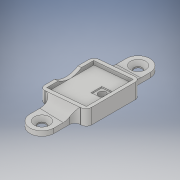
# Autodesk Inventor part: Kamerahalterung_Winkel_variabel
Saved by Autodesk Inventor 2019 (Build 230136000, 136)
## iProperties
Created: 2020-05-14
Part Number: Kamerahalterung_Winkel_variabel
Material: Generisch
Document SubType Name: Modeling
Designer: 111162002
Density: 1 g/cm^3
Appearance: Vorgabe
Author: 111162002
Autodesk Inventor part; units mm, degrees
ref_plane "YZ Plane" through (0, 0, 0) normal (1, 0, 0) x (0, 1, 0)
ref_plane "XZ Plane" through (0, 0, 0) normal (0, 1, 0) x (-1, 0, 0)
ref_plane "XY Plane" through (0, 0, 0) normal (0, 0, 1) x (1, 0, 0)
sketch "Skizze2" plane through (0, 0, 0) normal (0, 0, 1) x (1, 0, 0)
  line L0 (0, 0) -> (0, 9.3)
  line L1 (0, 9.3) -> (39, 12.7121)
  line L2 (39, 12.7121) -> (39, 0)
  line L3 (39, 0) -> (0, 0)
  dimension "d0" = 95
  dimension "d1" = 9.3
  dimension "d5" = 39
  constraints: 8 end point, 1 parallel, 1 perpendicular, 1 vertical
  measures "d0" angle of L1 L0
  measures "d1" distance of L0.start L0.end
  measures "d5" horizontal distance of L1.end L0.end
extrude "Extrusion1" add sketch "Skizze2" along normal blind 45
sketch "Skizze3" plane through (0, 9.3, 45) normal (-0.0871557, 0.9961947, 0) x (0.9961947, 0.0871557, 0)
  line L0 (3.0245, 42) -> (36.1245, 42)
  line L1 (36.1245, 42) -> (36.1245, 3)
  line L2 (36.1245, 3) -> (3.0245, 3)
  line L3 (3.0245, 3) -> (3.0245, 42)
  line L4 (39.149, 0) -> (0, 0) projected
  line L5 (39.149, 45) -> (39.149, 0) projected
  line L6 (33.249, 27.8623) -> (23.749, 27.8623)
  line L7 (23.749, 27.8623) -> (23.749, 18.8623)
  line L8 (23.749, 18.8623) -> (33.249, 18.8623)
  line L9 (33.249, 18.8623) -> (33.249, 27.8623)
  circle A0 centre (28.499, 23.3623) radius 3
  point P0 (-0.8105, 45)
  dimension "d6" = 39
  dimension "d7" = 33.1
  dimension "d8" = 3
  dimension "d9" = 3.0245
  dimension "d10" = 9
  dimension "d11" = 9.5
  dimension "d12" = 5.9
  dimension "d13" = 6
  dimension "d14" = 4.75
  constraints: 16 end point, 4 parallel, 2 horizontal, 2 perpendicular, 1 centre point
  measures "d6" distance of L0.end L1.end
  measures "d7" distance of L0.start L0.end
  measures "d8" distance between parallel lines of L4 L2
  measures "d9" distance between parallel lines of L5 L1
  measures "d10" distance of L6.end L7.end
  measures "d11" distance of L7.end L8.end
  measures "d12" distance between parallel lines of L5 L9
  measures "d13" diameter of A0
  measures "d14" distance from line of A0.centre L9
extrude "Extrusion2" cut sketch "Skizze3" against normal blind 3 contours L0 L1 L2 L3
extrude "Extrusion3" cut sketch "Skizze3" against normal up to surface contours A0 surface through (0, 0, 0) normal (0, -1, 0)
extrude "Extrusion4" cut sketch "Skizze3" against normal blind 4 contours L9 L8 L7 L6
sketch "Skizze5" plane through (0, 0, 0) normal (0, -1, 0) x (1, 0, 0)
  line L0 (39, 0) -> (0, 0) projected
  line L1 (9.5, 0) -> (29.5, 0)
  line L2 (29.5, 0) -> (29.5, -27.5)
  line L3 (29.5, -27.5) -> (9.5, -27.5)
  line L4 (9.5, -27.5) -> (9.5, 0)
  line L5 (0, 0) -> (0, 45) projected
  line L6 (0, 45) -> (39, 45) projected
  line L7 (9.5, 45) -> (29.5, 45)
  line L8 (29.5, 45) -> (29.5, 72.5)
  line L9 (29.5, 72.5) -> (9.5, 72.5)
  line L10 (9.5, 72.5) -> (9.5, 45)
  circle A0 centre (19.5, -17.5) radius 3.25
  circle A1 centre (19.5, 62.5) radius 3.25
  dimension "d26" = 20
  dimension "d27" = 9.5
  dimension "d28" = 27.5
  dimension "d29" = 27.5
  dimension "d30" = 20
  dimension "d32" = 9.5
  dimension "d35" = 6.5
  dimension "d36" = 6.5
  dimension "d37" = 10
  dimension "d38" = 10
  dimension "d39" = 10
  dimension "d40" = 10
  constraints: 16 end point, 4 parallel, 2 centre point, 2 horizontal, 2 perpendicular, 2 point on line
  measures "d26" distance of L2.end L3.end
  measures "d27" distance between parallel lines of L5 L4
  measures "d28" distance of L3.end L1.start
  measures "d29" distance of L9.end L7.start
  measures "d30" distance of L8.end L9.end
  measures "d32" distance between parallel lines of L5 L10
  measures "d35" diameter of A0
  measures "d36" diameter of A1
  measures "d37" distance from line of L2 A0.centre
  measures "d38" distance from line of L8 A1.centre
  measures "d39" distance from line of L3 A0.centre
  measures "d40" distance from line of L9 A1.centre
extrude "Extrusion7" add sketch "Skizze5" against normal blind 4
fillet "Rundung1" radius 4.5 8 edges at (0, 4.65, 45) (0, 4.65, 0) (9.5, 2, 0) (29.5, 2, 0) (39, 6.356, 0) (39, 6.356, 45) (29.5, 2, 45) (9.5, 2, 45)
fillet "Rundung2" radius 10 4 edges at (29.5, 2, -27.5) (9.5, 2, -27.5) (9.5, 2, 72.5) (29.5, 2, 72.5)
fillet "Rundung3" radius 10 6 edges at (7.25, 4, 0) (31.75, 4, 0) (19.5, 4, 0) (7.25, 4, 45) (31.75, 4, 45) (19.5, 4, 45)
fillet "Rundung4" [suppressed]
chamfer "Fase1" distance 3 angle 45 5 edges at (16.25, 4, 62.5) (16.25, 4, -17.5) (26.41, 0, 21.6377) (31.5785, 0, 23.7312) (31.5785, 0, 19.5443)
sketch "Skizze7" plane through (3.013, 9.5636, 42) normal (0.9961947, 0.0871557, 0) x (0, 0, -1)
  circle A0 centre (19.292, 14.25) radius 17.2
  line L0 (0, -3) -> (39, -3) projected
  point P0 (42, -9.2646)
  dimension "d54" = 34.4
  dimension "d55" = 17.25
  constraints: 1 centre point
  measures "d54" diameter of A0
  measures "d55" distance from line of L0 A0.centre
extrude "Extrusion9" cut sketch "Skizze7" against normal up to surface surface through (0, 9.3, 0) normal (-1, 0, 0)
